tablet attempt 1 (Autodesk Fusion 360 design; units mm, degrees)
Autodesk Fusion 360 part; units mm, degrees
sketch "bk" plane through (0, 0, 0) normal (0, 1, 0) x (1, 0, 0)
  line L0 (0, 0) -> (185, 0)
  line L1 (185, 0) -> (185, -115)
  line L2 (185, -115) -> (0, -115)
  line L3 (0, -115) -> (0, 0)
  line L4 (183, -113) -> (2, -113)
  line L5 (2, -113) -> (2, -2)
  line L6 (2, -2) -> (183, -2)
  line L7 (183, -2) -> (183, -113)
  dimension "d1" = 185
  dimension "d2" = 115
  dimension "d3" = 2
  constraint horizontal L0
  constraint vertical L1
  constraint horizontal L2
  constraint vertical L3
  constraint coincident L0.start L3.end
  measures "d1" distance of L0.start L0.end
  measures "d2" distance of L0.start L2.end
extrude "Extrude1" add sketch "bk" along normal blind 2.75 contours L0 L1 L2 L3 | L4 L5 L6 L7 makes body 1
extrude "Extrude1'" add sketch "bk" against normal blind 3.5 separate body makes body 2 in component "Component"
sketch "Sketch1" plane through (0, 2.75, 0) normal (0, 1, 0) x (-1, 0, 0) in component "Component"
  line L0 (0, 115) -> (-185, 115)
  line L1 (-185, 115) -> (-185, 0)
  line L2 (-185, 0) -> (0, 0)
  line L3 (0, 0) -> (0, 115)
  line L4 (3.7132, 61.0694) -> (3.7132, 47.7442) construction
  line L5 (3.7132, 47.7442) -> (13.7132, 47.7442) construction
  line L6 (13.7132, 47.7442) -> (13.7132, 61.0694) construction
  line L7 (13.7132, 61.0694) -> (3.7132, 61.0694) construction
  constraint perpendicular L4 L5
  constraint parallel L4 L6
  constraint parallel L5 L7
extrude "Extrude2" add 1 faces at (2, -1.1667, 76) along direction (1, 0, 0) blind 53 on bodies 2 bodies 2 in component "Component"
extrude "Extrude3" add 1 faces at (183, -1.1667, 39) along direction (-1, 0, 0) blind 21 on bodies 2 bodies 2 in component "Component"
sketch "Sketch2" plane through (0, -3.5, 0) normal (0, -1, 0) x (1, 0, 0) in component "Component"
  line L0 (162, 2) -> (55, 2)
  line L1 (55, 2) -> (55, 113)
  line L2 (55, 113) -> (162, 113)
  line L3 (162, 113) -> (162, 2)
  line L4 (185, 115) -> (0, 115)
  line L5 (0, 115) -> (0, 0)
  line L6 (0, 0) -> (185, 0)
  line L7 (185, 0) -> (185, 115)
  line L8 (-5, -5) -> (190, -5)
  line L9 (190, -5) -> (190, 120)
  line L10 (190, 120) -> (-5, 120)
  line L11 (-5, 120) -> (-5, -5)
  line L12 (-1, -1) -> (186, -1)
  line L13 (186, -1) -> (186, 116)
  line L14 (186, 116) -> (-1, 116)
  line L15 (-1, 116) -> (-1, -1)
  dimension "d12" = 5
  dimension "d13" = 1
extrude "Extrude4" add sketch "Sketch2" against normal blind 3.5 contours L8 L9 L10 L11 | L12 L13 L14 L15 bodies 2 in component "Component"
extrude "Extrude5" add sketch "Sketch2" against normal blind 7.5 contours L8 L9 L10 L11 bodies 2 in component "Component"
sketch "Sketch3" plane through (0, 0, 0) normal (0, 1, 0) x (1, 0, 0) in component "Component"
component "Component" placed x (1, 0, 0) y (0, 1, 0) z (0, 0, 1) at (0, 0, 0)
equation "d16 = -4.5 mm - 3 mm"
